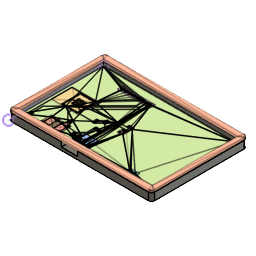
3d source file (Autodesk Fusion 360 design; units mm, degrees)
part number: 2026-06-07-18-30-23-417
Autodesk Fusion 360 part; units mm, degrees
sketch "Sketch1" plane through (0, 0, 0) normal (0, 1, 0) x (1, 0, 0)
  line L0 (0, 0) -> (94, 0)
  line L1 (94, 0) -> (94, 63)
  line L2 (94, 63) -> (0, 63)
  line L3 (0, 63) -> (0, 0)
  line L4 (90.5, 4) -> (2.5, 4)
  line L5 (2.5, 4) -> (2.5, 60)
  line L6 (2.5, 60) -> (90.5, 60)
  line L7 (90.5, 60) -> (90.5, 4)
  dimension "d3" = 63
  dimension "d4" = 94
  dimension "d5" = 56
  dimension "d6" = 88
  dimension "d7" = 2.5
  dimension "d8" = 3.5
  dimension "d9" = 3
  dimension "d10" = 4
  constraint horizontal L0
  constraint vertical L1
  constraint horizontal L2
  constraint vertical L3
  constraint coincident L0.start L3.end
  constraint horizontal L4
  constraint vertical L5
  constraint horizontal L6
  constraint vertical L7
  measures "d3" distance of L0.start L2.end
  measures "d4" distance of L1.end L2.end
  measures "d5" distance of L4.start L6.end
  measures "d6" distance of L4.start L4.end
  measures "d7" distance of L3 L5
  measures "d8" distance of L1 L7
  measures "d9" distance of L2 L6
  measures "d10" distance of L0 L4
sketch "Sketch2" plane through (0, 0, 0) normal (0, 1, 0) x (1, 0, 0)
  line L0 (0, 63) -> (0, 0)
  dimension "d11" = 63
  measures "d11" distance of L0.start L0.end
sketch "Sketch3" plane through (0, 0, 0) normal (0, 1, 0) x (1, 0, 0)
extrude "Extrude1" add sketch "Sketch1" along normal blind 5
sketch "Sketch4" plane through (0, 0, 0) normal (0, 1, 0) x (1, 0, 0)
  line L0 (2.4514, 59.9356) -> (90.5, 59.9356)
  line L1 (90.5, 59.9356) -> (90.5, 4)
  line L2 (90.5, 4) -> (2.4514, 4)
  line L3 (2.4514, 4) -> (2.4514, 59.9356)
  constraint horizontal L0
  constraint vertical L1
  constraint horizontal L2
  constraint vertical L3
extrude "Extrude2" add sketch "Sketch4" along normal blind 2
fillet "Fillet1" radius 2 4 edges at (94, 2.5, 0) (0, 2.5, 0) (94, 2.5, -63) (0, 2.5, -63)
other "Base Mesh Feature1"
sketch "Sketch5" plane through (0, 0, 0) normal (0, 1, 0) x (1, 0, 0)
other "CopyPasteMeshes1"
sketch "Sketch6" plane through (0, 0, 0) normal (0, 0, 1) x (1, 0, 0)
  line L0 (2, 5) -> (2, 0)
  line L1 (2, 0) -> (92, 0)
  line L2 (92, 0) -> (92, 5)
  line L3 (92, 5) -> (2, 5)
  line L4 (34.6717, 5) -> (45.3417, 5)
  line L5 (45.3417, 5) -> (45.3417, 0)
  line L6 (45.3417, 0) -> (34.6717, 0)
  line L7 (34.6717, 0) -> (34.6717, 5)
  dimension "d18" = 10.67
  constraint horizontal L4
  constraint vertical L5
  constraint horizontal L6
  constraint vertical L7
  constraint coincident L1 L5.end
  constraint coincident L3 L4.start
  measures "d18" distance of L4.start L4.end
extrude "Extrude3" cut sketch "Sketch6" along normal blind 0 and the other way blind 4 contours L1 L3 L4 L5 L6 L7
sketch "Sketch7" plane through (0, 0, -4) normal (0, 0, 1) x (1, 0, 0)
  line L0 (45.3417, 2) -> (34.6717, 2)
  line L1 (34.6717, 2) -> (34.6717, 0)
  line L2 (34.6717, 0) -> (45.3417, 0)
  line L3 (45.3417, 0) -> (45.3417, 2)
  line L4 (34.6717, 2) -> (45.3417, 2)
  line L5 (45.3417, 2) -> (45.3417, 0)
  line L6 (45.3417, 0) -> (34.6717, 0)
  line L7 (34.6717, 0) -> (34.6717, 2)
  constraint horizontal L4
  constraint vertical L5
  constraint horizontal L6
  constraint vertical L7
  constraint coincident L2.end L3.start
  constraint coincident L0.end L1.start
extrude "Extrude4" add sketch "Sketch7" along normal blind 4
other "Base Mesh Feature2"
